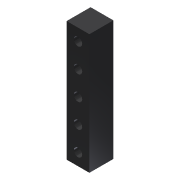
# Autodesk Inventor part: 5 pin header
Saved by Autodesk Inventor 2014 (Build 180170000, 170)
## iProperties
Created: 2015-11-19
Part Number: 5 pin header
Material: Generic
Document SubType Name: Modeling
Designer: Tom
Density: 1 g/cm^3
Appearance: Default
Author: Tom
Autodesk Inventor part; units mm, degrees
ref_plane "YZ Plane" through (0, 0, 0) normal (1, 0, 0) x (0, 1, 0)
ref_plane "XZ Plane" through (0, 0, 0) normal (0, 1, 0) x (-1, 0, 0)
ref_plane "XY Plane" through (0, 0, 0) normal (0, 0, 1) x (1, 0, 0)
sketch "Sketch1" plane through (0, 0, 0) normal (0, 0, 1) x (1, 0, 0)
  line L0 (0, 0) -> (2.413, 0)
  line L1 (2.413, 0) -> (2.413, 12.7)
  line L2 (2.413, 12.7) -> (0, 12.7)
  line L3 (0, 12.7) -> (0, 0)
  circle A0 centre (1.2065, 11.43) radius 0.4445
  circle A1 centre (1.2065, 8.89) radius 0.4445
  circle A2 centre (1.2065, 6.35) radius 0.4445
  circle A3 centre (1.2065, 3.81) radius 0.4445
  circle A4 centre (1.2065, 1.27) radius 0.4445
  dimension "d0" = 2.413
  dimension "d1" = 12.7
  dimension "d2" = 0.889
  dimension "d3" = 0.889
  dimension "d4" = 0.889
  dimension "d5" = 1.27
  dimension "d6" = 2.54
  dimension "d7" = 2.54
  dimension "d8" = 0.889
  dimension "d9" = 0.889
  dimension "d10" = 2.54
  dimension "d11" = 2.54
  dimension "d12" = 1.2065
  constraints: 8 end point, 5 centre point, 4 vertical alignment, 2 parallel, 1 horizontal, 1 perpendicular
  measures "d0" distance of L2.end L1.end
  measures "d1" distance of L1.end L0.end
  measures "d2" diameter of A0
  measures "d3" diameter of A1
  measures "d4" diameter of A2
  measures "d5" distance from line of L2 A0.centre
  measures "d6" distance of A0.centre A1.centre
  measures "d7" distance of A1.centre A2.centre
  measures "d8" diameter of A3
  measures "d9" diameter of A4
  measures "d10" distance of A2.centre A3.centre
  measures "d11" distance of A3.centre A4.centre
  measures "d12" horizontal distance of L1.end A0.centre
extrude "Extrusion1" add sketch "Sketch1" along normal blind 2.54
equation "\"d12\" = 0.5 * d0"
body "Solid1"
